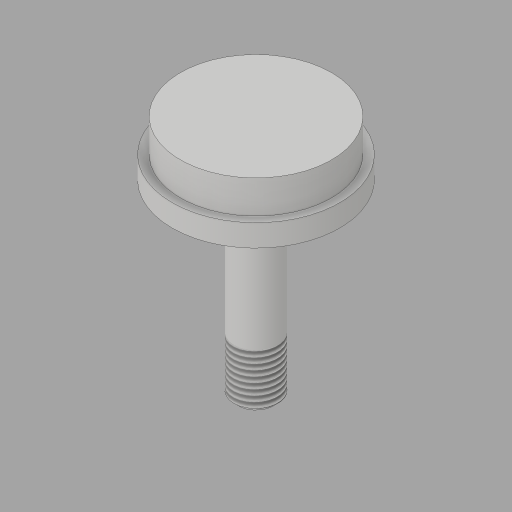
# Autodesk Inventor part: Rad Aufnahme
Saved by Autodesk Inventor 2023.2 (Build 272271000, 271)
## iProperties
Created: 2023-02-02
Part Number: Rad Aufnahme
Material: Generisch
Document SubType Name: Modeling
Designer: Raoul Messerli
Density: 1 g/cm^3
Appearance: Vorgabe
Author: Raoul Messerli
Autodesk Inventor part; units mm, degrees
ref_plane "YZ Plane" through (0, 0, 0) normal (1, 0, 0) x (0, 1, 0)
ref_plane "XZ Plane" through (0, 0, 0) normal (0, 1, 0) x (-1, 0, 0)
ref_plane "XY Plane" through (0, 0, 0) normal (0, 0, 1) x (1, 0, 0)
sketch "Skizze1" plane through (0, 0, 0) normal (1, 0, 0) x (0, 1, 0)
  line L0 (0, -29.1045) -> (0, 0)
  line L1 (0, 0) -> (0, -20.5338)
  line L2 (0, 0) -> (34.35, 0)
  line L3 (34.35, 0) -> (34.35, -15)
  line L4 (34.35, -15) -> (38.05, -15)
  line L5 (38.05, -15) -> (38.05, -25)
  line L6 (38.05, -25) -> (10, -25)
  line L7 (10, -25) -> (10, -110)
  line L8 (10, -110) -> (0, -110)
  line L9 (0, 0) -> (0, -24.283)
  line L10 (34.35, 0) -> (0, 0)
  line L11 (0, -132) -> (0, 22) projected
  line L12 (0, -110) -> (0, 0)
  dimension "d0" = 15
  dimension "d1" = 25
  dimension "d2" = 76.1
  dimension "d3" = 68.7
  dimension "d4" = 20
  dimension "d6" = 85
  constraints: 24 end point, 6 perpendicular, 4 point on line, 3 vertical, 1 collinear, 2 other
  measures "d0" distance between parallel lines of L4 L2
  measures "d1" distance between parallel lines of L6 L2
  measures "d2" diameter of L5 L0
  measures "d3" diameter of L3 L0
  measures "d4" diameter of L7 L0
  measures "d6" distance of L6.end L7.end
revolve "Umdrehung1" add sketch "Skizze1" angle 360 about axis through (0, 0, -110) along (0, 0, 1)
thread "Gewinde1" size "M20x2.5" class "6g" standard "ANSI Metric M Profile" length 25
chamfer "Fase1" distance 2 angle 45 1 edges at (0, -10, -110)
